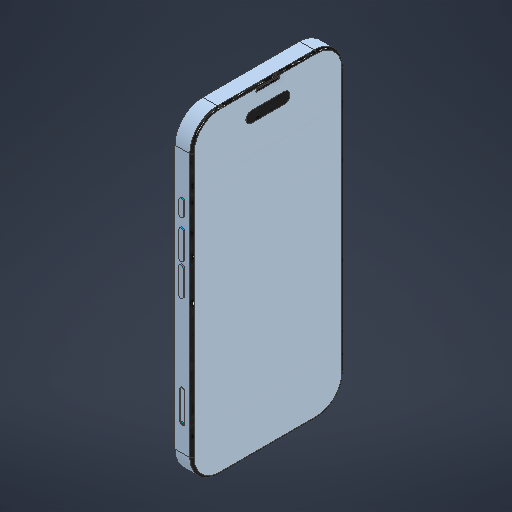
# Autodesk Inventor part: Iphone17
Saved by Autodesk Inventor 2027 (Build 310192060, 192F)
## iProperties
Created: 2026-09-24
Part Number: Iphone17
Material: Alumínio 6061-AHC
Document SubType Name: Modeling
Designer: labsfiap
Density: 2.7 g/cm^3
Appearance: Alumínio - Escuro
Author: labsfiap
Autodesk Inventor part; units mm, degrees
ref_plane "YZ Plane" through (0, 0, 0) normal (1, 0, 0) x (0, 1, 0)
ref_plane "XZ Plane" through (0, 0, 0) normal (0, 1, 0) x (-1, 0, 0)
ref_plane "XY Plane" through (0, 0, 0) normal (0, 0, 1) x (1, 0, 0)
sketch "Esboço1" plane through (0, 0, 0) normal (1, 0, 0) x (0, 1, 0)
  line L0 (0, 0) -> (149.6, 0)
  line L1 (149.6, 0) -> (149.6, -71.5)
  line L2 (149.6, -71.5) -> (0, -71.5)
  line L3 (0, -71.5) -> (0, 0)
  dimension "d0" = 149.6
  dimension "d1" = 71.5
  constraints: 8 end point, 3 perpendicular, 1 horizontal
  measures "d0" distance of L0.start L0.end
  measures "d1" distance of L0.end L1.end
extrude "Extrusão1" add sketch "Esboço1" along normal blind 7.95
fillet "Arredondamento1" radius 13 4 edges at (3.975, 149.6, -71.5) (3.975, 149.6, 0) (3.975, 0, 0) (3.975, 0, -71.5)
fillet "Arredondamento2" radius 1 8 edges at (7.95, 0, -35.75) (7.95, 3.8076, -67.6924) (7.95, 74.8, -71.5) (7.95, 145.7924, -67.6924) (7.95, 149.6, -35.75) (7.95, 145.7924, -3.8076) (7.95, 74.8, 0) (7.95, 3.8076, -3.8076)
sketch "Esboço2" plane through (0, 0, -58.5) normal (0, -1, 0) x (1, 0, 0)
  line L0 (6.95, 0) -> (0, 0) projected
  line L1 (0, 45.5) -> (6.95, 45.5) projected
  line L2 (3.475, 18.65) -> (4.775, 18.65)
  line L3 (4.775, 18.65) -> (2.175, 18.65)
  line L4 (2.175, 18.65) -> (2.175, 26.85)
  line L5 (2.175, 26.85) -> (4.775, 26.85)
  line L6 (4.775, 26.85) -> (4.775, 18.65)
  point P0 (0, 58.5)
  constraints: 10 end point, 3 perpendicular, 1 horizontal, 1 point on line
extrude "Extrusão2" cut sketch "Esboço2" against normal blind 6.2
fillet "Arredondamento3" radius 1.3 4 edges at (4.775, 3.1, -39.85) (2.175, 3.1, -39.85) (4.775, 3.1, -31.65) (2.175, 3.1, -31.65)
sketch "Esboço3" plane through (0, 6.2, -58.5) normal (0, -1, 0) x (1, 0, 0)
  arc A0 (4.775, 25.55) -> (2.175, 25.55) centre (3.475, 25.55) ccw projected
  arc A1 (2.175, 19.95) -> (4.775, 19.95) centre (3.475, 19.95) ccw projected
  line L0 (3.475, 25.55) -> (3.475, 19.95) construction
  line L1 (3.125, 25.55) -> (3.125, 19.95)
  line L2 (3.825, 19.95) -> (3.825, 25.55)
  arc A2 (3.825, 25.55) -> (3.125, 25.55) centre (3.475, 25.55) ccw
  arc A3 (3.125, 19.95) -> (3.825, 19.95) centre (3.475, 19.95) ccw
  point P0 (0, 58.5)
  point P1 (3.475, 22.75)
  constraints: 8 end point, 4 point on circle, 4 tangent, 2 centre point, 1 midpoint, 1 parallel
extrude "Extrusão3" add sketch "Esboço3" along normal blind 5.5
sketch "Esboço4" plane through (0, 0, 0) normal (-1, 0, 0) x (0, 0, 1)
  line L0 (-58.5, 149.6) -> (-13, 149.6) projected
  arc A0 (-58.5, 148.6) -> (-70.5, 136.6) centre (-58.5, 136.6) ccw projected
  line L1 (-66.5, 131.06) -> (-66.5, 110.31)
  line L2 (-45, 110.31) -> (-45, 131.06)
  arc A1 (-45, 131.06) -> (-66.5, 131.06) centre (-55.75, 131.06) ccw
  arc A2 (-66.5, 110.31) -> (-45, 110.31) centre (-55.75, 110.31) ccw
  circle A3 centre (-55.75, 131.06) radius 8.4
  circle A4 centre (-55.75, 131.06) radius 7.6
  circle A5 centre (-55.75, 131.06) radius 5.75
  circle A6 centre (-55.75, 110.31) radius 8.4
  circle A7 centre (-55.75, 110.31) radius 7.6
  circle A8 centre (-55.75, 110.31) radius 5.75
  point P0 (0, 0)
  constraints: 8 centre point, 6 coincident, 4 end point, 4 point on circle, 4 tangent, 1 parallel
extrude "Extrusão4" add sketch "Esboço4" along normal blind 2.2 contours A1 L2 A2 L1
sketch "Esboço5" plane through (0, 0, 0) normal (-1, 0, 0) x (0, 0, 1)
  circle A0 centre (-55.75, 131.06) radius 8.4 projected
  circle A1 centre (-55.75, 131.06) radius 7.6
  circle A2 centre (-55.75, 131.06) radius 5.75
  circle A3 centre (-55.75, 131.06) radius 8.4
  point P0 (0, 0)
  constraints: 3 centre point, 3 coincident, 1 concentric
extrude "Extrusão5" add sketch "Esboço5" along normal blind 3.3 contours A0
sketch "Esboço6" plane through (0, 131.06, -55.75) normal (-1, 0, 0) x (0, 0, 1)
  circle A0 centre (0, -20.75) radius 8.4 projected
  circle A1 centre (0, -20.75) radius 8.4
  circle A2 centre (0, -20.75) radius 7.6
  point P0 (55.75, -131.06)
  constraints: 2 centre point, 2 coincident
extrude "Extrusão6" add sketch "Esboço6" along normal blind 3.3
sketch "Esboço7" plane through (0, 131.06, -55.75) normal (-1, 0, 0) x (0, 0, 1)
  circle A0 centre (0, 0) radius 7.6
  circle A1 centre (0, -20.75) radius 7.6 projected
  circle A2 centre (0, -20.75) radius 7.6
  point P0 (55.75, -131.06)
  dimension "d38" = 15.2
  dimension "d40" = 15.2
  constraints: 2 centre point, 1 coincident
  measures "d38" diameter of A0
  measures "d40" diameter of A2
extrude "Extrusão7" add sketch "Esboço7" along normal blind 3.1
sketch "Esboço8" plane through (0, 0, 0) normal (-1, 0, 0) x (0, 0, 1)
  line L0 (-45, 110.31) -> (-45, 131.06) projected
  circle A0 centre (-35.7, 120.685) radius 2.5
  circle A1 centre (-35.7, 120.685) radius 2.3
  point P0 (0, 0)
  dimension "d45" = 4.6
  constraints: 2 centre point, 1 coincident
  measures "d45" diameter of A1
extrude "Extrusão8" add sketch "Esboço8" along normal blind 0.2 contours A0 | A1
sketch "Esboço9" plane through (0, 13, 0) normal (0, 0, 1) x (1, 0, 0)
  line L0 (0, 136.6) -> (6.95, 136.6) projected
  line L1 (2.375, 103) -> (2.375, 97.2)
  line L2 (4.575, 97.2) -> (4.575, 103)
  arc A0 (4.575, 103) -> (2.375, 103) centre (3.475, 103) ccw
  arc A1 (2.375, 97.2) -> (4.575, 97.2) centre (3.475, 97.2) ccw
  line L3 (3.475, 79.35) -> (3.475, 90.85) construction
  line L4 (4.575, 79.35) -> (4.575, 90.85)
  line L5 (2.375, 90.85) -> (2.375, 79.35)
  arc A2 (2.375, 79.35) -> (4.575, 79.35) centre (3.475, 79.35) ccw
  arc A3 (4.575, 90.85) -> (2.375, 90.85) centre (3.475, 90.85) ccw
  point P0 (0, -13)
  constraints: 12 end point, 8 point on circle, 8 tangent, 4 centre point, 2 parallel
sketch "Esboço10" plane through (0, 13, 0) normal (0, 0, 1) x (1, 0, 0)
  line L0 (3.4735, 64.3614) -> (3.4735, 75.8614) construction
  line L1 (4.5735, 64.3614) -> (4.5735, 75.8614)
  line L2 (2.3735, 75.8614) -> (2.3735, 64.3614)
  arc A0 (2.3735, 64.3614) -> (4.5735, 64.3614) centre (3.4735, 64.3614) ccw
  arc A1 (4.5735, 75.8614) -> (2.3735, 75.8614) centre (3.4735, 75.8614) ccw
  point P0 (0, -13)
  constraints: 8 end point, 4 point on circle, 4 tangent, 2 centre point, 1 parallel
extrude "Extrusão9" add sketch "Esboço9" along normal blind 0.6
extrude "Extrusão10" add sketch "Esboço10" along normal blind 0.65
sketch "Esboço11" plane through (0, 13, -71.5) normal (0, 0, -1) x (-1, 0, 0)
  line L0 (-6.95, 136.6) -> (0, 136.6) projected
  line L1 (0, 123.6) -> (-6.95, 123.6) projected
  line L2 (-6.95, 0) -> (0, 0) projected
  line L3 (-4.575, 84) -> (-4.575, 69.7)
  line L4 (-2.375, 69.7) -> (-2.375, 84)
  arc A0 (-2.375, 84) -> (-4.575, 84) centre (-3.475, 84) ccw
  arc A1 (-4.575, 69.7) -> (-2.375, 69.7) centre (-3.475, 69.7) ccw
  point P0 (0, -13)
  point P1 (-3.475, 76.85)
  constraints: 4 end point, 4 point on circle, 4 tangent, 2 centre point, 1 parallel
extrude "Extrusão11" add sketch "Esboço11" along normal blind 0.65
sketch "Esboço12" plane through (0, 13, -71.5) normal (0, 0, -1) x (-1, 0, 0)
  line L0 (-6.95, -13) -> (0, -13) projected
  arc A0 (-4.575, 69.7) -> (-2.375, 69.7) centre (-3.475, 69.7) ccw projected
  line L1 (-2.227, 37.3585) -> (-2.227, 51.5662)
  line L2 (-4.723, 51.5662) -> (-4.723, 37.3585)
  arc A1 (-4.723, 37.3585) -> (-2.227, 37.3585) centre (-3.475, 37.3585) ccw
  arc A2 (-2.227, 51.5662) -> (-4.723, 51.5662) centre (-3.475, 51.5662) ccw
  line L3 (-1.24, 37.335) -> (-1.24, 51.395)
  line L4 (-5.71, 51.395) -> (-5.71, 37.335)
  arc A3 (-5.71, 37.335) -> (-1.24, 37.335) centre (-3.475, 37.335) ccw
  arc A4 (-1.24, 51.395) -> (-5.71, 51.395) centre (-3.475, 51.395) ccw
  constraints: 8 end point, 8 point on circle, 8 tangent, 4 centre point, 2 parallel
extrude "Extrusão12" cut sketch "Esboço12" against normal blind 0.15 contours A1 L2 A2 L1 | A3 L4 A4 L3
fillet "Arredondamento4" radius 0.55 4 edges at (1.24, 57.365, -71.35) (3.475, 48.1, -71.35) (5.71, 57.365, -71.35) (3.475, 66.63, -71.35)
sketch "Esboço13" plane through (0, 13, -71.5) normal (0, 0, -1) x (-1, 0, 0)
  arc A0 (-1.6175, 51.395) -> (-5.3325, 51.395) centre (-3.475, 51.395) ccw projected
  line L0 (-4.575, 51.5927) -> (-4.575, 37.2627)
  line L1 (-2.375, 37.2627) -> (-2.375, 51.5927)
  arc A1 (-2.375, 51.5927) -> (-4.575, 51.5927) centre (-3.475, 51.5927) ccw
  arc A2 (-4.575, 37.2627) -> (-2.375, 37.2627) centre (-3.475, 37.2627) ccw
  point P0 (0, -13)
  constraints: 4 end point, 4 point on circle, 4 tangent, 2 centre point, 1 parallel
extrude "Extrusão13" add sketch "Esboço13" along normal blind 0.15
sketch "Esboço14" plane through (0, 13, 0) normal (0, 0, 1) x (1, 0, 0)
  line L0 (0, 136.6) -> (6.95, 136.6) projected
  line L1 (0, 0) -> (0, 123.6) projected
  line L2 (2.575, 25.7) -> (2.575, 12.5)
  line L3 (4.375, 12.5) -> (4.375, 25.7)
  arc A0 (4.375, 25.7) -> (2.575, 25.7) centre (3.475, 25.7) ccw
  arc A1 (2.575, 12.5) -> (4.375, 12.5) centre (3.475, 12.5) ccw
  circle A2 centre (3.475, 12.5) radius 0.5
  line L4 (2.325, 25.7) -> (2.325, 12.5)
  line L5 (4.625, 12.5) -> (4.625, 25.7)
  arc A3 (4.625, 25.7) -> (2.325, 25.7) centre (3.475, 25.7) ccw
  arc A4 (2.325, 12.5) -> (4.625, 12.5) centre (3.475, 12.5) ccw
  point P0 (0, -13)
  point P1 (3.475, 19.1)
  point P2 (3.475, 19.1)
  constraints: 8 end point, 8 point on circle, 8 tangent, 5 centre point, 2 parallel, 1 coincident
extrude "Extrusão14" cut sketch "Esboço14" against normal blind 0.01 contours A3 L5 A4 L4
sketch "Esboço15" plane through (3.475, 38.7, 0) normal (0, 0, 1) x (1, 0, 0)
  arc A0 (-0.9, -13.2) -> (0.9, -13.2) centre (0, -13.2) ccw projected
  circle A1 centre (0, -13.2) radius 0.5
  point P0 (-3.475, -38.7)
  constraints: 1 centre point, 1 coincident
extrude "Extrusão15" cut sketch "Esboço15" against normal blind 2.5
sketch "Esboço16" plane through (0, 0, -58.5) normal (0, -1, 0) x (1, 0, 0)
  line L0 (6.95, 45.5) -> (6.95, 58.5) projected
  line L1 (6.95, -13) -> (0, -13) projected
  line L2 (0, 20.3) -> (0, 25.3) projected
  circle A0 centre (3.475, 17.025) radius 1.05
  circle A1 centre (3.475, 17.025) radius 0.875
  circle A2 centre (3.475, 28.525) radius 1.05
  circle A3 centre (3.475, 28.525) radius 0.875
  line L3 (2.8591, 28.5571) -> (3.3152, 29.1207)
  line L4 (3.3152, 29.1207) -> (3.9921, 28.861)
  line L5 (3.9921, 28.861) -> (3.9544, 28.137)
  line L6 (3.9544, 28.137) -> (3.2541, 27.9492)
  line L7 (3.2541, 27.9492) -> (2.8591, 28.5571)
  line L8 (3.1031, 16.5131) -> (2.8732, 17.2205)
  line L9 (2.8732, 17.2205) -> (3.475, 17.6577)
  line L10 (3.475, 17.6577) -> (4.0768, 17.2205)
  line L11 (4.0768, 17.2205) -> (3.8469, 16.5131)
  line L12 (3.8469, 16.5131) -> (3.1031, 16.5131)
  point P0 (0, 58.5)
  constraints: 20 end point, 4 centre point, 4 coincident, 22 other
extrude "Extrusão16" cut sketch "Esboço16" against normal blind 0.2
fillet "Arredondamento5" radius 0.1 10 edges at (3.2541, 0.1, -30.5508) (3.9544, 0.1, -30.363) (3.9921, 0.1, -29.639) (3.3152, 0.1, -29.3793) (2.8591, 0.1, -29.9429) (3.1031, 0.1, -41.9869) (3.475, 0.1, -40.8423) (2.8732, 0.1, -41.2795) (3.8469, 0.1, -41.9869) (4.0768, 0.1, -41.2795)
sketch "Esboço17" plane through (0, 0, -58.5) normal (0, -1, 0) x (1, 0, 0)
  line L0 (6.95, 45.5) -> (6.95, 0) projected
  line L1 (6.95, 22.75) -> (0, 22.75)
  line L2 (0, 45.5) -> (0, 0) projected
  circle A0 centre (3.475, 13.3) radius 0.5
  circle A1 centre (3.475, 11.5) radius 0.5
  circle A2 centre (3.475, 9.7) radius 0.5
  circle A3 centre (3.475, 7.9) radius 0.5
  circle A4 centre (3.475, 6.1) radius 0.5
  circle A5 centre (3.475, 32.2) radius 0.5
  circle A6 centre (3.475, 34) radius 0.5
  circle A7 centre (3.475, 35.8) radius 0.5
  point P0 (0, 58.5)
  constraints: 8 centre point, 2 end point, 2 midpoint
extrude "Extrusão17" cut sketch "Esboço17" against normal blind 1.5
fillet "Arredondamento6" radius 2 4 edges at (0, 120.685, -45) (0, 99.56, -55.75) (0, 120.685, -66.5) (0, 141.81, -55.75)
sketch "Esboço18" plane through (-2.2, 0, 0) normal (-1, 0, 0) x (0, 0, 1)
  line L0 (-66.5, 110.31) -> (-66.5, 131.06) projected
  circle A0 centre (-46.7168, 120.685) radius 0.575
  point P0 (0, 0)
  constraints: 1 centre point
extrude "Extrusão18" cut sketch "Esboço18" against normal blind 1
sketch "Esboço19" plane through (7.95, 0, 0) normal (1, 0, 0) x (0, 0, -1)
  line L0 (13, 148.6) -> (58.5, 148.6) projected
  line L1 (30.15, 147) -> (41.35, 147)
  line L2 (30.15, 147) -> (30.15, 147.55)
  line L3 (30.15, 147.55) -> (30.15, 148.6)
  line L4 (41.35, 147) -> (41.35, 148.6)
  line L5 (30.15, 148.6) -> (41.35, 148.6)
  point P0 (0, 0)
  constraints: 10 end point, 3 point on line, 2 vertical, 1 perpendicular
extrude "Extrusão19" cut sketch "Esboço19" against normal blind 1
fillet "Arredondamento7" radius 0.275 2 edges at (7.45, 147, -30.15) (7.45, 147, -41.35)
sketch "Esboço20" plane through (7.95, 0, 0) normal (1, 0, 0) x (0, 0, -1)
  line L0 (30.15, 148.6) -> (41.35, 148.6) projected
  line L1 (27.97, 135.5) -> (43.53, 135.5)
  line L2 (43.53, 140.7) -> (27.97, 140.7)
  arc A0 (27.97, 140.7) -> (27.97, 135.5) centre (27.97, 138.1) ccw
  arc A1 (43.53, 135.5) -> (43.53, 140.7) centre (43.53, 138.1) ccw
  point P0 (0, 0)
  constraints: 4 end point, 4 point on circle, 4 tangent, 2 centre point, 1 parallel
extrude "Extrusão20" cut sketch "Esboço20" against normal blind 0.01
